Autodesk Fusion 360 part; units mm, degrees
note: some values were not read from the file. Chosen so that the rebuilt part matches the saved one: that a step has no effect.
(part 3 of 7)
  spline S620 degree 3 poles (-16.2697, 43.0639) (-16.2176, 42.4855) (-16.1655, 41.9071) (-16.1119, 41.3111) knots 0 0 0 0 1 1 1 1
  spline S621 degree 3 poles (-16.1119, 41.3111) (-16.0605, 39.9386) (-16.1203, 38.9907) (-16.5501, 37.7044) knots 0 0 0 0 1 1 1 1
  spline S622 degree 3 poles (-16.5501, 37.7044) (-16.8791, 37.7044) (-17.2082, 37.7044) (-17.5472, 37.7044) knots 0 0 0 0 1 1 1 1
  spline S623 degree 3 poles (-17.5472, 37.7044) (-17.5298, 37.2957) (-17.5125, 36.8869) (-17.4946, 36.4658) knots 0 0 0 0 1 1 1 1
  spline S624 degree 3 poles (-17.4946, 36.4658) (-17.4811, 35.9285) (-17.4676, 35.3912) (-17.4537, 34.8377) knots 0 0 0 0 1 1 1 1
  spline S625 degree 3 poles (-17.4537, 34.8377) (-17.4364, 34.3056) (-17.419, 33.7734) (-17.4011, 33.2252) knots 0 0 0 0 1 1 1 1
  spline S626 degree 3 poles (-17.4011, 33.2252) (-17.5472, 31.7217) (-17.5472, 31.7217) (-19.0429, 29.7275) knots 0 0 0 0 1 1 1 1
  spline S627 degree 3 poles (-19.0429, 29.7275) (-17.3976, 29.7275) (-15.7524, 29.7275) (-14.0573, 29.7275) knots 0 0 0 0 1 1 1 1
  spline S628 degree 3 poles (-14.0573, 29.7275) (-14.0573, 30.0565) (-14.0573, 30.3856) (-14.0573, 30.7246) knots 0 0 0 0 1 1 1 1
  spline S629 degree 3 poles (-14.0573, 30.7246) (-13.5637, 30.7246) (-13.0702, 30.7246) (-12.5616, 30.7246) knots 0 0 0 0 1 1 1 1
  spline S630 degree 3 poles (-12.5616, 30.7246) (-12.3971, 31.2182) (-12.2326, 31.7117) (-12.0631, 32.2203) knots 0 0 0 0 1 1 1 1
  spline S631 degree 3 poles (-12.0631, 32.2203) (-11.8725, 31.3946) (-11.7071, 30.5628) (-11.5645, 29.7275) knots 0 0 0 0 1 1 1 1
  spline S632 degree 3 poles (-11.5645, 29.7275) (-12.0631, 29.2289) (-12.0631, 29.2289) (-13.8567, 29.1803) knots 0 0 0 0 1 1 1 1
  spline S633 degree 3 poles (-13.8567, 29.1803) (-14.5987, 29.1836) (-15.3407, 29.1895) (-16.0827, 29.1978) knots 0 0 0 0 1 1 1 1
  spline S634 degree 3 poles (-16.0827, 29.1978) (-16.65, 29.2012) (-16.65, 29.2012) (-17.2288, 29.2046) knots 0 0 0 0 1 1 1 1
  spline S635 degree 3 poles (-17.2288, 29.2046) (-18.1659, 29.2105) (-19.1029, 29.2194) (-20.04, 29.2289) knots 0 0 0 0 1 1 1 1
  spline S636 degree 3 poles (-20.04, 29.2289) (-20.2868, 29.9693) (-20.2868, 29.9693) (-20.5385, 30.7246) knots 0 0 0 0 1 1 1 1
  spline S637 degree 3 poles (-20.5385, 30.7246) (-20.374, 31.0537) (-20.2095, 31.3827) (-20.04, 31.7217) knots 0 0 0 0 1 1 1 1
  spline S638 degree 3 poles (-20.04, 31.7217) (-19.7109, 31.7217) (-19.3819, 31.7217) (-19.0429, 31.7217) knots 0 0 0 0 1 1 1 1
  spline S639 degree 3 poles (-19.0429, 31.7217) (-18.3848, 36.4929) (-17.7267, 41.2641) (-17.0486, 46.1798) knots 0 0 0 0 1 1 1 1
  spline S640 degree 3 poles (-38.9851, 32.7188) (-37.998, 32.3898) (-37.0108, 32.0607) (-35.9938, 31.7217) knots 0 0 0 0 1 1 1 1
  spline S641 degree 3 poles (-35.9938, 31.7217) (-35.9938, 31.3927) (-35.9938, 31.0636) (-35.9938, 30.7246) knots 0 0 0 0 1 1 1 1
  spline S642 degree 3 poles (-35.9938, 30.7246) (-35.3357, 31.0537) (-34.6776, 31.3827) (-33.9995, 31.7217) knots 0 0 0 0 1 1 1 1
  spline S643 degree 3 poles (-33.9995, 31.7217) (-33.9995, 32.0508) (-33.9995, 32.3798) (-33.9995, 32.7188) knots 0 0 0 0 1 1 1 1
  spline S644 degree 3 poles (-33.9995, 32.7188) (-33.506, 32.7188) (-33.0124, 32.7188) (-32.5039, 32.7188) knots 0 0 0 0 1 1 1 1
  spline S645 degree 3 poles (-32.5039, 32.7188) (-32.3394, 32.3898) (-32.1748, 32.0607) (-32.0053, 31.7217) knots 0 0 0 0 1 1 1 1
  spline S646 degree 3 poles (-32.0053, 31.7217) (-30.5246, 31.7217) (-29.0439, 31.7217) (-27.5183, 31.7217) knots 0 0 0 0 1 1 1 1
  spline S647 degree 3 poles (-27.5183, 31.7217) (-27.3538, 31.0636) (-27.1893, 30.4055) (-27.0198, 29.7275) knots 0 0 0 0 1 1 1 1
  spline S648 degree 3 poles (-27.0198, 29.7275) (-30.4911, 28.562) (-33.1588, 28.6348) (-36.4923, 30.2261) knots 0 0 0 0 1 1 1 1
  spline S649 degree 3 poles (-36.4923, 30.2261) (-37.5065, 30.9946) (-38.1768, 31.7219) (-38.9851, 32.7188) knots 0 0 0 0 1 1 1 1
  spline S650 degree 3 poles (-5.0833, -7.6642) (-5.0833, -7.9933) (-5.0833, -8.3223) (-5.0833, -8.6613) knots 0 0 0 0 1 1 1 1
  spline S651 degree 3 poles (-5.0833, -8.6613) (-4.2607, -8.8258) (-3.4381, -8.9904) (-2.5905, -9.1599) knots 0 0 0 0 1 1 1 1
  spline S652 degree 3 poles (-2.5905, -9.1599) (-2.9196, -9.9825) (-3.2486, -10.8051) (-3.5876, -11.6527) knots 0 0 0 0 1 1 1 1
  spline S653 degree 3 poles (-3.5876, -11.6527) (-3.9, -11.6829) (-4.2123, -11.7131) (-4.5341, -11.7442) knots 0 0 0 0 1 1 1 1
  spline S654 degree 3 poles (-4.5341, -11.7442) (-4.9416, -11.786) (-5.349, -11.8277) (-5.7688, -11.8708) knots 0 0 0 0 1 1 1 1
  spline S655 degree 3 poles (-5.7688, -11.8708) (-6.1737, -11.9113) (-6.5786, -11.9517) (-6.9957, -11.9935) knots 0 0 0 0 1 1 1 1
  spline S656 degree 3 poles (-6.9957, -11.9935) (-8.0959, -12.0968) (-8.0959, -12.0968) (-9.0717, -12.6498) knots 0 0 0 0 1 1 1 1
  spline S657 degree 3 poles (-9.0717, -12.6498) (-9.4008, -12.3207) (-9.7298, -11.9917) (-10.0689, -11.6527) knots 0 0 0 0 1 1 1 1
  spline S658 degree 3 poles (-10.0689, -11.6527) (-8.8515, -8.8526) (-8.8515, -8.8526) (-7.5761, -7.9758) knots 0 0 0 0 1 1 1 1
  spline S659 degree 3 poles (-7.5761, -7.9758) (-6.579, -7.6642) (-6.579, -7.6642) (-5.0833, -7.6642) knots 0 0 0 0 1 1 1 1
  spline S660 degree 3 poles (-5.5819, 0.8112) (-5.471, 0.363) (-5.471, 0.363) (-5.3579, -0.0943) knots 0 0 0 0 1 1 1 1
  spline S661 degree 3 poles (-5.3579, -0.0943) (-5.1425, -0.9483) (-4.913, -1.7987) (-4.6782, -2.6475) knots 0 0 0 0 1 1 1 1
  spline S662 degree 3 poles (-4.6782, -2.6475) (-4.5847, -4.1743) (-4.5847, -4.1743) (-5.5195, -5.5453) knots 0 0 0 0 1 1 1 1
  spline S663 degree 3 poles (-5.5195, -5.5453) (-5.8692, -5.9155) (-6.2188, -6.2857) (-6.579, -6.6671) knots 0 0 0 0 1 1 1 1
  spline S664 degree 3 poles (-6.579, -6.6671) (-6.7435, -6.9961) (-6.908, -7.3252) (-7.0775, -7.6642) knots 0 0 0 0 1 1 1 1
  spline S665 degree 3 poles (-7.0775, -7.6642) (-8.3259, -8.0888) (-8.3259, -8.0888) (-9.8507, -8.4744) knots 0 0 0 0 1 1 1 1
  spline S666 degree 3 poles (-9.8507, -8.4744) (-10.3552, -8.6042) (-10.8597, -8.734) (-11.3795, -8.8678) knots 0 0 0 0 1 1 1 1
  spline S667 degree 3 poles (-11.3795, -8.8678) (-11.7696, -8.9642) (-12.1597, -9.0606) (-12.5616, -9.1599) knots 0 0 0 0 1 1 1 1
  spline S668 degree 3 poles (-12.5616, -9.1599) (-12.5616, -8.8308) (-12.5616, -8.5018) (-12.5616, -8.1628) knots 0 0 0 0 1 1 1 1
  spline S669 degree 3 poles (-12.5616, -8.1628) (-12.8907, -8.1628) (-13.2197, -8.1628) (-13.5588, -8.1628) knots 0 0 0 0 1 1 1 1
  spline S670 degree 3 poles (-13.5588, -8.1628) (-14.1196, -5.2961) (-14.1196, -5.2961) (-13.5588, -4.1743) knots 0 0 0 0 1 1 1 1
  spline S671 degree 3 poles (-13.5588, -4.1743) (-13.2297, -4.1743) (-12.9007, -4.1743) (-12.5616, -4.1743) knots 0 0 0 0 1 1 1 1
  spline S672 degree 3 poles (-12.5616, -4.1743) (-12.5616, -3.3517) (-12.5616, -2.5291) (-12.5616, -1.6815) knots 0 0 0 0 1 1 1 1
  spline S673 degree 3 poles (-12.5616, -1.6815) (-12.2326, -1.6815) (-11.9035, -1.6815) (-11.5645, -1.6815) knots 0 0 0 0 1 1 1 1
  spline S674 degree 3 poles (-11.5645, -1.6815) (-11.7291, -3.4913) (-11.8936, -5.301) (-12.0631, -7.1656) knots 0 0 0 0 1 1 1 1
  spline S675 degree 3 poles (-12.0631, -7.1656) (-10.5992, -7.8313) (-10.5992, -7.8313) (-9.3152, -7.1715) knots 0 0 0 0 1 1 1 1
  spline S676 degree 3 poles (-9.3152, -7.1715) (-7.7171, -5.8795) (-7.2541, -4.4864) (-6.6724, -2.5852) knots 0 0 0 0 1 1 1 1
  spline S677 degree 3 poles (-6.6724, -2.5852) (-6.5648, -2.259) (-6.4572, -1.9329) (-6.3462, -1.5968) knots 0 0 0 0 1 1 1 1
  spline S678 degree 3 poles (-6.3462, -1.5968) (-6.0834, -0.7967) (-5.8315, 0.007) (-5.5819, 0.8112) knots 0 0 0 0 1 1 1 1
  spline S679 degree 3 poles (24.3296, 14.9831) (26.0233, 14.6232) (26.8004, 13.6084) (27.8214, 12.278) knots 0 0 0 0 1 1 1 1
  spline S680 degree 3 poles (27.8214, 12.278) (28.5444, 10.1089) (28.5619, 8.1594) (27.946, 5.9526) knots 0 0 0 0 1 1 1 1
  spline S681 degree 3 poles (27.946, 5.9526) (26.9552, 4.1196) (26.0218, 3.0365) (24.0199, 2.3692) knots 0 0 0 0 1 1 1 1
  spline S682 degree 3 poles (24.0199, 2.3692) (23.6292, 2.3487) (23.2384, 2.3281) (22.8358, 2.3069) knots 0 0 0 0 1 1 1 1
  spline S683 degree 3 poles (22.8358, 2.3069) (22.5068, 2.636) (22.1777, 2.965) (21.8387, 3.304) knots 0 0 0 0 1 1 1 1
  spline S684 degree 3 poles (21.8387, 3.304) (22.6613, 3.304) (23.484, 3.304) (24.3315, 3.304) knots 0 0 0 0 1 1 1 1
  spline S685 degree 3 poles (24.3315, 3.304) (24.3624, 3.6125) (24.3932, 3.921) (24.425, 4.2388) knots 0 0 0 0 1 1 1 1
  spline S686 degree 3 poles (24.425, 4.2388) (24.5587, 4.5884) (24.6923, 4.938) (24.8301, 5.2983) knots 0 0 0 0 1 1 1 1
  spline S687 degree 3 poles (24.8301, 5.2983) (26.1018, 5.863) (26.1018, 5.863) (27.3228, 6.2954) knots 0 0 0 0 1 1 1 1
  spline S688 degree 3 poles (27.3228, 6.2954) (27.2795, 7.1891) (27.2256, 8.0823) (27.167, 8.9751) knots 0 0 0 0 1 1 1 1
  spline S689 degree 3 poles (27.167, 8.9751) (27.1237, 9.7212) (27.1237, 9.7212) (27.0794, 10.4825) knots 0 0 0 0 1 1 1 1
  spline S690 degree 3 poles (27.0794, 10.4825) (26.9952, 10.9105) (26.911, 11.3385) (26.8243, 11.7795) knots 0 0 0 0 1 1 1 1
  spline S691 degree 3 poles (26.8243, 11.7795) (26.3307, 12.1085) (25.8371, 12.4376) (25.3286, 12.7766) knots 0 0 0 0 1 1 1 1
  spline S692 degree 3 poles (25.3286, 12.7766) (25.3286, 13.1056) (25.3286, 13.4347) (25.3286, 13.7737) knots 0 0 0 0 1 1 1 1
  spline S693 degree 3 poles (25.3286, 13.7737) (24.835, 13.6092) (24.3415, 13.4447) (23.8329, 13.2751) knots 0 0 0 0 1 1 1 1
  spline S694 degree 3 poles (23.8329, 13.2751) (23.1378, 13.2419) (22.4411, 13.2326) (21.7452, 13.244) knots 0 0 0 0 1 1 1 1
  spline S695 degree 3 poles (21.7452, 13.244) (20.8044, 13.2594) (20.8044, 13.2594) (19.8445, 13.2751) knots 0 0 0 0 1 1 1 1
  spline S696 degree 3 poles (19.8445, 13.2751) (20.9861, 14.9876) (22.3538, 15.0522) (24.3296, 14.9831) knots 0 0 0 0 1 1 1 1
  spline S697 degree 3 poles (-31.5068, 15.2694) (-31.1777, 15.2694) (-30.8487, 15.2694) (-30.5097, 15.2694) knots 0 0 0 0 1 1 1 1
  spline S698 degree 3 poles (-30.5097, 15.2694) (-30.5097, 14.4468) (-30.5097, 13.6241) (-30.5097, 12.7766) knots 0 0 0 0 1 1 1 1
  spline S699 degree 3 poles (-30.5097, 12.7766) (-30.2012, 12.9411) (-29.8927, 13.1056) (-29.5749, 13.2751) knots 0 0 0 0 1 1 1 1
  spline S700 degree 3 poles (-29.5749, 13.2751) (-26.8442, 14.149) (-24.1154, 14.2507) (-21.4733, 13.0882) knots 0 0 0 0 1 1 1 1
  spline S701 degree 3 poles (-21.4733, 13.0882) (-21.1648, 12.8208) (-20.8564, 12.5535) (-20.5385, 12.278) knots 0 0 0 0 1 1 1 1
  spline S702 degree 3 poles (-20.5385, 12.278) (-20.5385, 11.949) (-20.5385, 11.6199) (-20.5385, 11.2809) knots 0 0 0 0 1 1 1 1
  spline S703 degree 3 poles (-20.5385, 11.2809) (-21.0321, 11.1164) (-21.5257, 10.9519) (-22.0342, 10.7824) knots 0 0 0 0 1 1 1 1
  spline S704 degree 3 poles (-22.0342, 10.7824) (-22.0342, 11.1114) (-22.0342, 11.4405) (-22.0342, 11.7795) knots 0 0 0 0 1 1 1 1
  spline S705 degree 3 poles (-22.0342, 11.7795) (-25.4087, 11.8301) (-28.6666, 11.7946) (-32.0053, 11.2809) knots 0 0 0 0 1 1 1 1
  spline S706 degree 3 poles (-32.0053, 11.2809) (-32.4693, 12.5801) (-32.5783, 13.0967) (-32.0365, 14.3969) knots 0 0 0 0 1 1 1 1
  spline S707 degree 3 poles (-32.0365, 14.3969) (-31.8617, 14.6848) (-31.6869, 14.9727) (-31.5068, 15.2694) knots 0 0 0 0 1 1 1 1
  spline S708 degree 3 poles (-28.0792, 48.7661) (-27.5663, 48.7732) (-27.0535, 48.7802) (-26.5251, 48.7875) knots 0 0 0 0 1 1 1 1
  spline S709 degree 3 poles (-26.5251, 48.7875) (-24.9983, 48.6705) (-23.9125, 48.3196) (-22.5328, 47.6755) knots 0 0 0 0 1 1 1 1
  spline S710 degree 3 poles (-22.5328, 47.6755) (-24.1968, 47.1208) (-24.4136, 47.2732) (-26.0227, 47.6755) knots 0 0 0 0 1 1 1 1
  spline S711 degree 3 poles (-26.0227, 47.6755) (-27.1858, 47.6949) (-28.3495, 47.6979) (-29.5125, 47.6755) knots 0 0 0 0 1 1 1 1
  spline S712 degree 3 poles (-29.5125, 47.6755) (-29.5125, 47.511) (-29.5125, 47.3465) (-29.5125, 47.177) knots 0 0 0 0 1 1 1 1
  spline S713 degree 3 poles (-29.5125, 47.177) (-28.3609, 46.8479) (-27.2092, 46.5189) (-26.0227, 46.1798) knots 0 0 0 0 1 1 1 1
  spline S714 degree 3 poles (-26.0227, 46.1798) (-26.0227, 46.0153) (-26.0227, 45.8508) (-26.0227, 45.6813) knots 0 0 0 0 1 1 1 1
  spline S715 degree 3 poles (-26.0227, 45.6813) (-26.335, 45.6684) (-26.6473, 45.6556) (-26.9691, 45.6423) knots 0 0 0 0 1 1 1 1
  spline S716 degree 3 poles (-26.9691, 45.6423) (-27.3766, 45.6141) (-27.784, 45.5858) (-28.2038, 45.5566) knots 0 0 0 0 1 1 1 1
  spline S717 degree 3 poles (-28.2038, 45.5566) (-28.6087, 45.5335) (-29.0136, 45.5104) (-29.4308, 45.4865) knots 0 0 0 0 1 1 1 1
  spline S718 degree 3 poles (-29.4308, 45.4865) (-30.5867, 45.289) (-30.5867, 45.289) (-31.1173, 44.2479) knots 0 0 0 0 1 1 1 1
  spline S719 degree 3 poles (-31.1173, 44.2479) (-31.2458, 43.8983) (-31.3743, 43.5487) (-31.5068, 43.1885) knots 0 0 0 0 1 1 1 1
  spline S720 degree 3 poles (-31.5068, 43.1885) (-31.6919, 42.7361) (-31.8769, 42.2836) (-32.0676, 41.8175) knots 0 0 0 0 1 1 1 1
  spline S721 degree 3 poles (-32.0676, 41.8175) (-32.2116, 41.4473) (-32.3556, 41.0771) (-32.5039, 40.6957) knots 0 0 0 0 1 1 1 1
  spline S722 degree 3 poles (-32.5039, 40.6957) (-33.096, 42.4055) (-32.9039, 43.3769) (-32.2858, 45.0581) knots 0 0 0 0 1 1 1 1
  spline S723 degree 3 poles (-32.2858, 45.0581) (-32.1424, 45.4565) (-31.9991, 45.855) (-31.8515, 46.2655) knots 0 0 0 0 1 1 1 1
  spline S724 degree 3 poles (-31.8515, 46.2655) (-31.6808, 46.7167) (-31.6808, 46.7167) (-31.5068, 47.177) knots 0 0 0 0 1 1 1 1
  spline S725 degree 3 poles (-31.5068, 47.177) (-32.4939, 47.0124) (-33.4811, 46.8479) (-34.4981, 46.6784) knots 0 0 0 0 1 1 1 1
  spline S726 degree 3 poles (-34.4981, 46.6784) (-32.3504, 48.3817) (-30.8035, 48.7491) (-28.0792, 48.7661) knots 0 0 0 0 1 1 1 1
  spline S727 degree 3 poles (-73.3855, 16.2665) (-72.6376, 15.581) (-72.6376, 15.581) (-71.8898, 14.7708) knots 0 0 0 0 1 1 1 1
  spline S728 degree 3 poles (-71.8898, 14.7708) (-71.8898, 14.4418) (-71.8898, 14.1127) (-71.8898, 13.7737) knots 0 0 0 0 1 1 1 1
  spline S729 degree 3 poles (-71.8898, 13.7737) (-72.2189, 13.7737) (-72.5479, 13.7737) (-72.8869, 13.7737) knots 0 0 0 0 1 1 1 1
  spline S730 degree 3 poles (-72.8869, 13.7737) (-72.964, 13.3418) (-72.964, 13.3418) (-73.0427, 12.9012) knots 0 0 0 0 1 1 1 1
  spline S731 degree 3 poles (-73.0427, 12.9012) (-73.4398, 11.6017) (-73.9791, 10.7956) (-74.8811, 9.7853) knots 0 0 0 0 1 1 1 1
  spline S732 degree 3 poles (-74.8811, 9.7853) (-75.2102, 9.7853) (-75.5392, 9.7853) (-75.8783, 9.7853) knots 0 0 0 0 1 1 1 1
  spline S733 degree 3 poles (-75.8783, 9.7853) (-75.8783, 8.9626) (-75.8783, 8.14) (-75.8783, 7.2925) knots 0 0 0 0 1 1 1 1
  spline S734 degree 3 poles (-75.8783, 7.2925) (-76.2073, 7.2925) (-76.5363, 7.2925) (-76.8754, 7.2925) knots 0 0 0 0 1 1 1 1
  spline S735 degree 3 poles (-76.8754, 7.2925) (-77.2044, 6.3053) (-77.5335, 5.3182) (-77.8725, 4.3011) knots 0 0 0 0 1 1 1 1
  spline S736 degree 3 poles (-77.8725, 4.3011) (-78.8054, 6.7198) (-77.5957, 8.5127) (-76.6164, 10.7512) knots 0 0 0 0 1 1 1 1
  spline S737 degree 3 poles (-76.6164, 10.7512) (-75.6728, 12.703) (-74.5953, 14.469) (-73.3855, 16.2665) knots 0 0 0 0 1 1 1 1
  spline S738 degree 3 poles (47.2651, -7.6642) (48.418, -7.5396) (48.418, -7.5396) (49.7579, -7.6642) knots 0 0 0 0 1 1 1 1
  spline S739 degree 3 poles (49.7579, -7.6642) (50.7238, -8.5055) (50.7238, -8.5055) (51.2535, -9.6584) knots 0 0 0 0 1 1 1 1
  spline S740 degree 3 poles (51.2535, -9.6584) (50.9731, -10.9983) (50.9731, -10.9983) (50.2564, -12.1512) knots 0 0 0 0 1 1 1 1
  spline S741 degree 3 poles (50.2564, -12.1512) (49.3216, -12.6809) (49.3216, -12.6809) (48.2622, -12.6498) knots 0 0 0 0 1 1 1 1
  spline S742 degree 3 poles (48.2622, -12.6498) (47.1404, -11.6838) (47.1404, -11.6838) (46.268, -10.6555) knots 0 0 0 0 1 1 1 1
  spline S743 degree 3 poles (46.268, -10.6555) (46.597, -9.6684) (46.9261, -8.6813) (47.2651, -7.6642) knots 0 0 0 0 1 1 1 1
  spline S744 degree 3 poles (-57.8854, 16.8799) (-56.9331, 16.765) (-56.9331, 16.765) (-55.936, 15.7679) knots 0 0 0 0 1 1 1 1
  spline S745 degree 3 poles (-55.936, 15.7679) (-55.8737, 14.4592) (-55.8737, 14.4592) (-55.936, 13.2751) knots 0 0 0 0 1 1 1 1
  spline S746 degree 3 poles (-55.936, 13.2751) (-57.0877, 13.1106) (-58.2393, 12.9461) (-59.4259, 12.7766) knots 0 0 0 0 1 1 1 1
  spline S747 degree 3 poles (-59.4259, 12.7766) (-59.2614, 13.2702) (-59.0969, 13.7637) (-58.9274, 14.2723) knots 0 0 0 0 1 1 1 1
  spline S748 degree 3 poles (-58.9274, 14.2723) (-59.75, 14.4368) (-60.5726, 14.6013) (-61.4201, 14.7708) knots 0 0 0 0 1 1 1 1
  spline S749 degree 3 poles (-61.4201, 14.7708) (-61.4201, 14.4418) (-61.4201, 14.1127) (-61.4201, 13.7737) knots 0 0 0 0 1 1 1 1
  spline S750 degree 3 poles (-61.4201, 13.7737) (-61.7492, 13.7737) (-62.0782, 13.7737) (-62.4172, 13.7737) knots 0 0 0 0 1 1 1 1
  spline S751 degree 3 poles (-62.4172, 13.7737) (-61.2918, 16.6998) (-61.1108, 16.8156) (-57.8854, 16.8799) knots 0 0 0 0 1 1 1 1
  spline S752 degree 3 poles (-67.4028, 18.7593) (-66.9092, 18.5947) (-66.4157, 18.4302) (-65.9071, 18.2607) knots 0 0 0 0 1 1 1 1
  spline S753 degree 3 poles (-65.9071, 18.2607) (-66.4817, 16.7286) (-67.146, 15.2847) (-67.9014, 13.836) knots 0 0 0 0 1 1 1 1
  spline S754 degree 3 poles (-67.9014, 13.836) (-69.616, 10.4196) (-70.1059, 7.0736) (-70.3941, 3.304) knots 0 0 0 0 1 1 1 1
  spline S755 degree 3 poles (-70.3941, 3.304) (-70.7232, 3.304) (-71.0522, 3.304) (-71.3913, 3.304) knots 0 0 0 0 1 1 1 1
  spline S756 degree 3 poles (-71.3913, 3.304) (-71.4952, 6.4979) (-71.4702, 9.2517) (-70.3941, 12.278) knots 0 0 0 0 1 1 1 1
  spline S757 degree 3 poles (-70.3941, 12.278) (-70.0651, 12.278) (-69.736, 12.278) (-69.397, 12.278) knots 0 0 0 0 1 1 1 1
  spline S758 degree 3 poles (-69.397, 12.278) (-69.4073, 12.6482) (-69.4176, 13.0184) (-69.4282, 13.3998) knots 0 0 0 0 1 1 1 1
  spline S759 degree 3 poles (-69.4282, 13.3998) (-69.4004, 14.6236) (-69.244, 15.599) (-68.8985, 16.765) knots 0 0 0 0 1 1 1 1
  spline S760 degree 3 poles (-68.8985, 16.765) (-68.4049, 16.765) (-67.9113, 16.765) (-67.4028, 16.765) knots 0 0 0 0 1 1 1 1
  spline S761 degree 3 poles (-67.4028, 16.765) (-67.4028, 17.4231) (-67.4028, 18.0812) (-67.4028, 18.7593) knots 0 0 0 0 1 1 1 1
  spline S762 degree 3 poles (-20.5385, 11.2809) (-20.374, 11.2809) (-20.2095, 11.2809) (-20.04, 11.2809) knots 0 0 0 0 1 1 1 1
  spline S763 degree 3 poles (-20.04, 11.2809) (-19.8618, 8.0442) (-20.4392, 5.5886) (-21.5356, 2.5562) knots 0 0 0 0 1 1 1 1
  spline S764 degree 3 poles (-21.5356, 2.5562) (-21.6783, 2.1462) (-21.821, 1.7361) (-21.968, 1.3137) knots 0 0 0 0 1 1 1 1
  spline S765 degree 3 poles (-21.968, 1.3137) (-22.3169, 0.3134) (-22.6734, -0.6844) (-23.0313, -1.6815) knots 0 0 0 0 1 1 1 1
  spline S766 degree 3 poles (-23.0313, -1.6815) (-24.0284, -0.6844) (-24.0284, -0.6844) (-24.1219, 0.7489) knots 0 0 0 0 1 1 1 1
  spline S767 degree 3 poles (-24.1219, 0.7489) (-24.0454, 2.024) (-23.9032, 3.0879) (-23.5299, 4.3011) knots 0 0 0 0 1 1 1 1
  spline S768 degree 3 poles (-23.5299, 4.3011) (-23.2008, 4.3011) (-22.8718, 4.3011) (-22.5328, 4.3011) knots 0 0 0 0 1 1 1 1
  spline S769 degree 3 poles (-22.5328, 4.3011) (-22.4711, 4.8667) (-22.4094, 5.4322) (-22.3458, 6.0149) knots 0 0 0 0 1 1 1 1
  spline S770 degree 3 poles (-22.3458, 6.0149) (-22.243, 6.601) (-22.1401, 7.1872) (-22.0342, 7.791) knots 0 0 0 0 1 1 1 1
  spline S771 degree 3 poles (-22.0342, 7.791) (-21.7052, 7.9556) (-21.3761, 8.1201) (-21.0371, 8.2896) knots 0 0 0 0 1 1 1 1
  spline S772 degree 3 poles (-21.0371, 8.2896) (-21.0474, 8.6906) (-21.0577, 9.0916) (-21.0683, 9.5048) knots 0 0 0 0 1 1 1 1
  spline S773 degree 3 poles (-21.0683, 9.5048) (-21.0371, 10.7824) (-21.0371, 10.7824) (-20.5385, 11.2809) knots 0 0 0 0 1 1 1 1
  spline S774 degree 3 poles (25.8272, 48.6726) (26.3207, 48.3436) (26.8143, 48.0145) (27.3228, 47.6755) knots 0 0 0 0 1 1 1 1
  spline S775 degree 3 poles (27.3228, 47.6755) (25.5131, 47.511) (23.7033, 47.3465) (21.8387, 47.177) knots 0 0 0 0 1 1 1 1
  spline S776 degree 3 poles (21.8387, 47.177) (23.0726, 46.6834) (23.0726, 46.6834) (24.3315, 46.1798) knots 0 0 0 0 1 1 1 1
  spline S777 degree 3 poles (24.3315, 46.1798) (24.3315, 46.0153) (24.3315, 45.8508) (24.3315, 45.6813) knots 0 0 0 0 1 1 1 1
  spline S778 degree 3 poles (24.3315, 45.6813) (23.3253, 45.4541) (22.3191, 45.2269) (21.3129, 44.9997) knots 0 0 0 0 1 1 1 1
  spline S779 degree 3 poles (21.3129, 44.9997) (20.2398, 44.7317) (20.2398, 44.7317) (19.3459, 43.6871) knots 0 0 0 0 1 1 1 1
  spline S780 degree 3 poles (19.3459, 43.6871) (19.3459, 44.3452) (19.3459, 45.0033) (19.3459, 45.6813) knots 0 0 0 0 1 1 1 1
  spline S781 degree 3 poles (19.3459, 45.6813) (19.8395, 45.6813) (20.3331, 45.6813) (20.8416, 45.6813) knots 0 0 0 0 1 1 1 1
  spline S782 degree 3 poles (20.8416, 45.6813) (20.2293, 46.5017) (20.2293, 46.5017) (19.3459, 47.177) knots 0 0 0 0 1 1 1 1
  spline S783 degree 3 poles (19.3459, 47.177) (18.317, 47.0132) (18.317, 47.0132) (17.3517, 46.6784) knots 0 0 0 0 1 1 1 1
  spline S784 degree 3 poles (17.3517, 46.6784) (17.0227, 46.8429) (16.6936, 47.0074) (16.3546, 47.177) knots 0 0 0 0 1 1 1 1
  spline S785 degree 3 poles (16.3546, 47.177) (19.2337, 49.1512) (22.4334, 49.0215) (25.8272, 48.6726) knots 0 0 0 0 1 1 1 1
  spline S786 degree 3 poles (-63.9129, 23.7448) (-63.5839, 23.2513) (-63.2548, 22.7577) (-62.9158, 22.2492) knots 0 0 0 0 1 1 1 1
  spline S787 degree 3 poles (-62.9158, 22.2492) (-63.3065, 21.8687) (-63.6973, 21.4882) (-64.0999, 21.0962) knots 0 0 0 0 1 1 1 1
  spline S788 degree 3 poles (-64.0999, 21.0962) (-65.4448, 19.8018) (-65.4448, 19.8018) (-66.4057, 18.2607) knots 0 0 0 0 1 1 1 1
  spline S789 degree 3 poles (-66.4057, 18.2607) (-66.7347, 18.4252) (-67.0638, 18.5898) (-67.4028, 18.7593) knots 0 0 0 0 1 1 1 1
  spline S790 degree 3 poles (-67.4028, 18.7593) (-67.5673, 18.2657) (-67.7318, 17.7721) (-67.9014, 17.2636) knots 0 0 0 0 1 1 1 1
  spline S791 degree 3 poles (-67.9014, 17.2636) (-68.0659, 17.5926) (-68.2304, 17.9217) (-68.3999, 18.2607) knots 0 0 0 0 1 1 1 1
  spline S792 degree 3 poles (-68.3999, 18.2607) (-68.729, 18.4252) (-69.058, 18.5898) (-69.397, 18.7593) knots 0 0 0 0 1 1 1 1
  spline S793 degree 3 poles (-69.397, 18.7593) (-68.7738, 20.2238) (-68.7738, 20.2238) (-67.9014, 21.7506) knots 0 0 0 0 1 1 1 1
  spline S794 degree 3 poles (-67.9014, 21.7506) (-66.9354, 22.0934) (-66.9354, 22.0934) (-65.9071, 22.2492) knots 0 0 0 0 1 1 1 1
  spline S795 degree 3 poles (-65.9071, 22.2492) (-64.8067, 22.991) (-64.8067, 22.991) (-63.9129, 23.7448) knots 0 0 0 0 1 1 1 1
  spline S796 degree 3 poles (-23.8103, 26.8296) (-21.8826, 26.7282) (-20.1085, 26.3788) (-18.2288, 25.9572) knots 0 0 0 0 1 1 1 1
  spline S797 degree 3 poles (-18.2288, 25.9572) (-16.9218, 25.6786) (-16.9218, 25.6786) (-15.0544, 25.739) knots 0 0 0 0 1 1 1 1
  spline S798 degree 3 poles (-15.0544, 25.739) (-15.0544, 25.41) (-15.0544, 25.081) (-15.0544, 24.7419) knots 0 0 0 0 1 1 1 1
  spline S799 degree 3 poles (-15.0544, 24.7419) (-16.2697, 24.7285) (-17.4848, 24.7186) (-18.7001, 24.7108) knots 0 0 0 0 1 1 1 1
  spline S800 degree 3 poles (-18.7001, 24.7108) (-19.0443, 24.7066) (-19.3884, 24.7024) (-19.743, 24.6981) knots 0 0 0 0 1 1 1 1
  spline S801 degree 3 poles (-19.743, 24.6981) (-21.3105, 24.6905) (-22.5299, 24.741) (-24.0284, 25.2405) knots 0 0 0 0 1 1 1 1
  spline S802 degree 3 poles (-24.0284, 25.2405) (-24.0284, 24.7469) (-24.0284, 24.2534) (-24.0284, 23.7448) knots 0 0 0 0 1 1 1 1
  spline S803 degree 3 poles (-24.0284, 23.7448) (-23.6994, 23.7448) (-23.3703, 23.7448) (-23.0313, 23.7448) knots 0 0 0 0 1 1 1 1
  spline S804 degree 3 poles (-23.0313, 23.7448) (-23.0313, 23.4158) (-23.0313, 23.0867) (-23.0313, 22.7477) knots 0 0 0 0 1 1 1 1
  spline S805 degree 3 poles (-23.0313, 22.7477) (-24.2652, 23.2413) (-24.2652, 23.2413) (-25.5241, 23.7448) knots 0 0 0 0 1 1 1 1
  spline S806 degree 3 poles (-25.5241, 23.7448) (-25.5454, 24.5755) (-25.5444, 25.4069) (-25.5241, 26.2376) knots 0 0 0 0 1 1 1 1
  spline S807 degree 3 poles (-25.5241, 26.2376) (-25.0255, 26.7362) (-25.0255, 26.7362) (-23.8103, 26.8296) knots 0 0 0 0 1 1 1 1
  spline S808 degree 3 poles (-45.4663, 24.7419) (-43.3459, 22.7889) (-42.1288, 21.316) (-41.844, 18.4009) knots 0 0 0 0 1 1 1 1
  spline S809 degree 3 poles (-41.844, 18.4009) (-41.8466, 17.9433) (-41.8492, 17.4858) (-41.8518, 17.0143) knots 0 0 0 0 1 1 1 1
  spline S810 degree 3 poles (-41.8518, 17.0143) (-41.8492, 16.5567) (-41.8467, 16.0992) (-41.844, 15.6277) knots 0 0 0 0 1 1 1 1
  spline S811 degree 3 poles (-41.844, 15.6277) (-41.9851, 14.1836) (-42.3735, 13.0938) (-42.9736, 11.7795) knots 0 0 0 0 1 1 1 1
  spline S812 degree 3 poles (-42.9736, 11.7795) (-43.1381, 11.7795) (-43.3026, 11.7795) (-43.4721, 11.7795) knots 0 0 0 0 1 1 1 1
  spline S813 degree 3 poles (-43.4721, 11.7795) (-43.4855, 12.8389) (-43.4952, 13.8983) (-43.5033, 14.9578) knots 0 0 0 0 1 1 1 1
  spline S814 degree 3 poles (-43.5033, 14.9578) (-43.5091, 15.5477) (-43.5148, 16.1377) (-43.5208, 16.7456) knots 0 0 0 0 1 1 1 1
  spline S815 degree 3 poles (-43.5208, 16.7456) (-43.4721, 18.2607) (-43.4721, 18.2607) (-42.9736, 19.2578) knots 0 0 0 0 1 1 1 1
  spline S816 degree 3 poles (-42.9736, 19.2578) (-43.2101, 19.556) (-43.4466, 19.8542) (-43.6902, 20.1615) knots 0 0 0 0 1 1 1 1
  spline S817 degree 3 poles (-43.6902, 20.1615) (-44.4692, 21.252) (-44.4692, 21.252) (-44.9678, 22.7477) knots 0 0 0 0 1 1 1 1
  spline S818 degree 3 poles (-44.9678, 22.7477) (-45.4614, 22.5832) (-45.9549, 22.4187) (-46.4635, 22.2492) knots 0 0 0 0 1 1 1 1
  spline S819 degree 3 poles (-46.4635, 22.2492) (-46.628, 22.5782) (-46.7925, 22.9072) (-46.962, 23.2463) knots 0 0 0 0 1 1 1 1
  spline S820 degree 3 poles (-46.962, 23.2463) (-46.633, 23.2463) (-46.3039, 23.2463) (-45.9649, 23.2463) knots 0 0 0 0 1 1 1 1
  spline S821 degree 3 poles (-45.9649, 23.2463) (-45.8004, 23.7398) (-45.6358, 24.2334) (-45.4663, 24.7419) knots 0 0 0 0 1 1 1 1
  spline S822 degree 3 poles (-24.0284, 25.2405) (-21.067, 25.076) (-18.1056, 24.9114) (-15.0544, 24.7419) knots 0 0 0 0 1 1 1 1
  spline S823 degree 3 poles (-15.0544, 24.7419) (-17.0486, 22.7477) (-17.0486, 22.7477) (-18.5521, 22.553) knots 0 0 0 0 1 1 1 1
  spline S824 degree 3 poles (-18.5521, 22.553) (-19.0842, 22.5761) (-19.6164, 22.5992) (-20.1646, 22.6231) knots 0 0 0 0 1 1 1 1
  spline S825 degree 3 poles (-20.1646, 22.6231) (-20.7019, 22.6411) (-21.2392, 22.6591) (-21.7927, 22.6776) knots 0 0 0 0 1 1 1 1
  spline S826 degree 3 poles (-21.7927, 22.6776) (-22.2015, 22.7007) (-22.6102, 22.7239) (-23.0313, 22.7477) knots 0 0 0 0 1 1 1 1
  spline S827 degree 3 poles (-23.0313, 22.7477) (-23.0313, 23.0768) (-23.0313, 23.4058) (-23.0313, 23.7448) knots 0 0 0 0 1 1 1 1
  spline S828 degree 3 poles (-23.0313, 23.7448) (-23.3604, 23.7448) (-23.6894, 23.7448) (-24.0284, 23.7448) knots 0 0 0 0 1 1 1 1
  spline S829 degree 3 poles (-24.0284, 23.7448) (-24.0284, 24.2384) (-24.0284, 24.732) (-24.0284, 25.2405) knots 0 0 0 0 1 1 1 1
  spline S830 degree 3 poles (31.8098, 33.2174) (34.081, 32.9404) (34.081, 32.9404) (34.8012, 32.2203) knots 0 0 0 0 1 1 1 1
  spline S831 degree 3 poles (34.8012, 32.2203) (34.9258, 31.005) (34.9258, 31.005) (34.8012, 29.7275) knots 0 0 0 0 1 1 1 1
  spline S832 degree 3 poles (34.8012, 29.7275) (33.3055, 28.7304) (33.3055, 28.7304) (32.2772, 28.855) knots 0 0 0 0 1 1 1 1
  spline S833 degree 3 poles (32.2772, 28.855) (31.3113, 29.2289) (31.3113, 29.2289) (30.3142, 30.2261) knots 0 0 0 0 1 1 1 1
  spline S834 degree 3 poles (30.3142, 30.2261) (30.4971, 31.6891) (30.7451, 32.1527) (31.8098, 33.2174) knots 0 0 0 0 1 1 1 1
  spline S835 degree 3 poles (-27.5183, 25.2405) (-27.6828, 24.7469) (-27.8474, 24.2534) (-28.0169, 23.7448) knots 0 0 0 0 1 1 1 1
  spline S836 degree 3 poles (-28.0169, 23.7448) (-28.0169, 24.0739) (-28.0169, 24.4029) (-28.0169, 24.7419) knots 0 0 0 0 1 1 1 1
  spline S837 degree 3 poles (-28.0169, 24.7419) (-29.532, 24.4813) (-29.532, 24.4813) (-30.6655, 23.4955) knots 0 0 0 0 1 1 1 1
  spline S838 degree 3 poles (-30.6655, 23.4955) (-31.9543, 22.3499) (-33.3255, 22.4068) (-34.9967, 22.2492) knots 0 0 0 0 1 1 1 1
  spline S839 degree 3 poles (-34.9967, 22.2492) (-35.1612, 21.7556) (-35.3257, 21.262) (-35.4952, 20.7535) knots 0 0 0 0 1 1 1 1
  spline S840 degree 3 poles (-35.4952, 20.7535) (-35.9888, 20.7535) (-36.4824, 20.7535) (-36.9909, 20.7535) knots 0 0 0 0 1 1 1 1
  spline S841 degree 3 poles (-36.9909, 20.7535) (-36.9909, 21.5761) (-36.9909, 22.3987) (-36.9909, 23.2463) knots 0 0 0 0 1 1 1 1
  spline S842 degree 3 poles (-36.9909, 23.2463) (-35.6941, 23.6775) (-34.3959, 24.1024) (-33.0959, 24.5238) knots 0 0 0 0 1 1 1 1
  spline S843 degree 3 poles (-33.0959, 24.5238) (-32.728, 24.6469) (-32.3601, 24.77) (-31.981, 24.8968) knots 0 0 0 0 1 1 1 1
  spline S844 degree 3 poles (-31.981, 24.8968) (-29.1834, 25.7955) (-29.1834, 25.7955) (-27.5183, 25.2405) knots 0 0 0 0 1 1 1 1
  spline S845 degree 3 poles (51.2535, 14.7708) (50.9817, 11.2375) (49.9527, 8.1261) (48.7607, 4.7997) knots 0 0 0 0 1 1 1 1
  spline S846 degree 3 poles (48.7607, 4.7997) (48.5946, 5.4644) (48.4284, 6.1292) (48.2622, 6.7939) knots 0 0 0 0 1 1 1 1
  spline S847 degree 3 poles (48.2622, 6.7939) (48.1549, 7.1101) (48.0475, 7.4263) (47.937, 7.7521) knots 0 0 0 0 1 1 1 1
  spline S848 degree 3 poles (47.937, 7.7521) (47.7047, 9.1407) (48.0429, 10.0758) (48.4803, 11.4056) knots 0 0 0 0 1 1 1 1
  spline S849 degree 3 poles (48.4803, 11.4056) (48.6236, 11.8503) (48.7669, 12.295) (48.9146, 12.7532) knots 0 0 0 0 1 1 1 1
  spline S850 degree 3 poles (48.9146, 12.7532) (49.0284, 13.09) (49.1421, 13.4267) (49.2593, 13.7737) knots 0 0 0 0 1 1 1 1
  spline S851 degree 3 poles (49.2593, 13.7737) (48.9303, 13.9382) (48.6012, 14.1028) (48.2622, 14.2723) knots 0 0 0 0 1 1 1 1
  spline S852 degree 3 poles (48.2622, 14.2723) (49.7579, 14.7708) (49.7579, 14.7708) (51.2535, 14.7708) knots 0 0 0 0 1 1 1 1
  spline S853 degree 3 poles (-44.4692, 11.7795) (-44.1402, 11.7795) (-43.8111, 11.7795) (-43.4721, 11.7795) knots 0 0 0 0 1 1 1 1
  spline S854 degree 3 poles (-43.4721, 11.7795) (-44.316, 8.5916) (-46.8333, 6.9576) (-49.5483, 5.3606) knots 0 0 0 0 1 1 1 1
  spline S855 degree 3 poles (-49.5483, 5.3606) (-50.9505, 4.7997) (-50.9505, 4.7997) (-52.9447, 4.7997) knots 0 0 0 0 1 1 1 1
  spline S856 degree 3 poles (-52.9447, 4.7997) (-52.9447, 5.1287) (-52.9447, 5.4578) (-52.9447, 5.7968) knots 0 0 0 0 1 1 1 1
  spline S857 degree 3 poles (-52.9447, 5.7968) (-51.9575, 5.7968) (-50.9704, 5.7968) (-49.9533, 5.7968) knots 0 0 0 0 1 1 1 1
  spline S858 degree 3 poles (-49.9533, 5.7968) (-49.9533, 6.1259) (-49.9533, 6.4549) (-49.9533, 6.7939) knots 0 0 0 0 1 1 1 1
  spline S859 degree 3 poles (-49.9533, 6.7939) (-49.6243, 6.9584) (-49.2952, 7.123) (-48.9562, 7.2925) knots 0 0 0 0 1 1 1 1
  spline S860 degree 3 poles (-48.9562, 7.2925) (-48.9562, 7.786) (-48.9562, 8.2796) (-48.9562, 8.7881) knots 0 0 0 0 1 1 1 1
  spline S861 degree 3 poles (-48.9562, 8.7881) (-48.6272, 8.7881) (-48.2981, 8.7881) (-47.9591, 8.7881) knots 0 0 0 0 1 1 1 1
  spline S862 degree 3 poles (-47.9591, 8.7881) (-47.7946, 9.1172) (-47.6301, 9.4462) (-47.4606, 9.7853) knots 0 0 0 0 1 1 1 1
  spline S863 degree 3 poles (-47.4606, 9.7853) (-46.4193, 10.1212) (-45.5642, 10.2838) (-44.4692, 10.2838) knots 0 0 0 0 1 1 1 1
  spline S864 degree 3 poles (-44.4692, 10.2838) (-44.4692, 10.7774) (-44.4692, 11.271) (-44.4692, 11.7795) knots 0 0 0 0 1 1 1 1
  spline S865 degree 3 poles (-45.9649, -7.6642) (-45.6358, -8.1578) (-45.3068, -8.6513) (-44.9678, -9.1599) knots 0 0 0 0 1 1 1 1
  spline S866 degree 3 poles (-44.9678, -9.1599) (-45.4614, -9.4067) (-45.4614, -9.4067) (-45.9649, -9.6584) knots 0 0 0 0 1 1 1 1
  spline S867 degree 3 poles (-45.9649, -9.6584) (-46.0369, -9.9875) (-46.1089, -10.3165) (-46.183, -10.6555) knots 0 0 0 0 1 1 1 1
  spline S868 degree 3 poles (-46.183, -10.6555) (-46.2756, -10.9846) (-46.3681, -11.3136) (-46.4635, -11.6527) knots 0 0 0 0 1 1 1 1
  spline S869 degree 3 poles (-46.4635, -11.6527) (-46.957, -11.8172) (-47.4506, -11.9817) (-47.9591, -12.1512) knots 0 0 0 0 1 1 1 1
  spline S870 degree 3 poles (-47.9591, -12.1512) (-48.1236, -12.4803) (-48.2882, -12.8093) (-48.4577, -13.1483) knots 0 0 0 0 1 1 1 1
  spline S871 degree 3 poles (-48.4577, -13.1483) (-45.1672, -13.1483) (-41.8767, -13.1483) (-38.4866, -13.1483) knots 0 0 0 0 1 1 1 1
  spline S872 degree 3 poles (-38.4866, -13.1483) (-38.6511, -11.6676) (-38.8156, -10.1869) (-38.9851, -8.6613) knots 0 0 0 0 1 1 1 1
  spline S873 degree 3 poles (-38.9851, -8.6613) (-38.8206, -8.6613) (-38.6561, -8.6613) (-38.4866, -8.6613) knots 0 0 0 0 1 1 1 1
  spline S874 degree 3 poles (-38.4866, -8.6613) (-38.3065, -9.3979) (-38.1307, -10.1356) (-37.9568, -10.8737) knots 0 0 0 0 1 1 1 1
  spline S875 degree 3 poles (-37.9568, -10.8737) (-37.8093, -11.4897) (-37.8093, -11.4897) (-37.6589, -12.1181) knots 0 0 0 0 1 1 1 1
  spline S876 degree 3 poles (-37.6589, -12.1181) (-37.603, -12.4581) (-37.547, -12.798) (-37.4894, -13.1483) knots 0 0 0 0 1 1 1 1
  spline S877 degree 3 poles (-37.4894, -13.1483) (-37.988, -13.6469) (-37.988, -13.6469) (-39.0514, -13.7035) knots 0 0 0 0 1 1 1 1
  spline S878 degree 3 poles (-39.0514, -13.7035) (-39.5083, -13.7009) (-39.9652, -13.6983) (-40.436, -13.6956) knots 0 0 0 0 1 1 1 1
  spline S879 degree 3 poles (-40.436, -13.6956) (-40.9292, -13.694) (-41.4225, -13.6924) (-41.9307, -13.6907) knots 0 0 0 0 1 1 1 1
  spline S880 degree 3 poles (-41.9307, -13.6907) (-42.4496, -13.6865) (-42.9686, -13.6823) (-43.5033, -13.678) knots 0 0 0 0 1 1 1 1
  spline S881 degree 3 poles (-43.5033, -13.678) (-44.0242, -13.6758) (-44.545, -13.6735) (-45.0817, -13.6712) knots 0 0 0 0 1 1 1 1
  spline S882 degree 3 poles (-45.0817, -13.6712) (-46.3732, -13.6653) (-47.6647, -13.6571) (-48.9562, -13.6469) knots 0 0 0 0 1 1 1 1
  spline S883 degree 3 poles (-48.9562, -13.6469) (-48.9562, -11.4659) (-48.7549, -11.1517) (-47.4606, -9.5338) knots 0 0 0 0 1 1 1 1
  spline S884 degree 3 poles (-47.4606, -9.5338) (-47.1829, -9.1816) (-46.9053, -8.8294) (-46.6192, -8.4666) knots 0 0 0 0 1 1 1 1
  spline S885 degree 3 poles (-46.6192, -8.4666) (-46.4033, -8.2018) (-46.1874, -7.937) (-45.9649, -7.6642) knots 0 0 0 0 1 1 1 1
  spline S886 degree 3 poles (-30.0111, 24.7419) (-29.353, 24.7419) (-28.6949, 24.7419) (-28.0169, 24.7419) knots 0 0 0 0 1 1 1 1
  spline S887 degree 3 poles (-28.0169, 24.7419) (-28.074, 24.0248) (-28.1376, 23.3082) (-28.2038, 22.5919) knots 0 0 0 0 1 1 1 1
  spline S888 degree 3 poles (-28.2038, 22.5919) (-28.2385, 22.1928) (-28.2732, 21.7937) (-28.309, 21.3825) knots 0 0 0 0 1 1 1 1
  spline S889 degree 3 poles (-28.309, 21.3825) (-28.5154, 20.2549) (-28.5154, 20.2549) (-29.5125, 18.7593) knots 0 0 0 0 1 1 1 1
  spline S890 degree 3 poles (-29.5125, 18.7593) (-29.5125, 19.2528) (-29.5125, 19.7464) (-29.5125, 20.2549) knots 0 0 0 0 1 1 1 1
  spline S891 degree 3 poles (-29.5125, 20.2549) (-30.3352, 20.4195) (-31.1578, 20.584) (-32.0053, 20.7535) knots 0 0 0 0 1 1 1 1
  spline S892 degree 3 poles (-32.0053, 20.7535) (-31.8408, 21.5761) (-31.6763, 22.3987) (-31.5068, 23.2463) knots 0 0 0 0 1 1 1 1
  spline S893 degree 3 poles (-31.5068, 23.2463) (-31.1777, 23.2463) (-30.8487, 23.2463) (-30.5097, 23.2463) knots 0 0 0 0 1 1 1 1
  spline S894 degree 3 poles (-30.5097, 23.2463) (-30.3451, 23.7398) (-30.1806, 24.2334) (-30.0111, 24.7419) knots 0 0 0 0 1 1 1 1
  spline S895 degree 3 poles (7.8792, 42.1914) (8.0437, 42.1914) (8.2082, 42.1914) (8.3777, 42.1914) knots 0 0 0 0 1 1 1 1
  spline S896 degree 3 poles (8.3777, 42.1914) (8.0794, 38.1995) (7.756, 34.2115) (7.3806, 30.2261) knots 0 0 0 0 1 1 1 1
  spline S897 degree 3 poles (7.3806, 30.2261) (6.3935, 30.5551) (5.4063, 30.8841) (4.3893, 31.2232) knots 0 0 0 0 1 1 1 1
  spline S898 degree 3 poles (4.3893, 31.2232) (4.6132, 31.962) (4.8427, 32.6992) (5.0748, 33.4355) knots 0 0 0 0 1 1 1 1
  spline S899 degree 3 poles (5.0748, 33.4355) (5.202, 33.8462) (5.3293, 34.2568) (5.4604, 34.6799) knots 0 0 0 0 1 1 1 1
  spline S900 degree 3 poles (5.4604, 34.6799) (5.8849, 35.7102) (5.8849, 35.7102) (6.882, 36.2087) knots 0 0 0 0 1 1 1 1
  spline S901 degree 3 poles (6.882, 36.2087) (7.2272, 37.6096) (7.2272, 37.6096) (7.4429, 39.2312) knots 0 0 0 0 1 1 1 1
  spline S902 degree 3 poles (7.4429, 39.2312) (7.5265, 39.782) (7.61, 40.3328) (7.6961, 40.9002) knots 0 0 0 0 1 1 1 1
  spline S903 degree 3 poles (7.6961, 40.9002) (7.7565, 41.3263) (7.8169, 41.7524) (7.8792, 42.1914) knots 0 0 0 0 1 1 1 1
  spline S904 degree 3 poles (-29.014, 5.7968) (-28.8495, 5.7968) (-28.6849, 5.7968) (-28.5154, 5.7968) knots 0 0 0 0 1 1 1 1
  spline S905 degree 3 poles (-28.5154, 5.7968) (-28.9168, 2.7868) (-29.4551, -0.1922) (-30.0111, -3.1772) knots 0 0 0 0 1 1 1 1
  spline S906 degree 3 poles (-30.0111, -3.1772) (-30.3401, -3.1772) (-30.6692, -3.1772) (-31.0082, -3.1772) knots 0 0 0 0 1 1 1 1
  spline S907 degree 3 poles (-31.0082, -3.1772) (-30.9774, -3.7222) (-30.9465, -4.2672) (-30.9147, -4.8287) knots 0 0 0 0 1 1 1 1
  spline S908 degree 3 poles (-30.9147, -4.8287) (-31.0082, -6.6671) (-31.0082, -6.6671) (-31.6937, -7.5707) knots 0 0 0 0 1 1 1 1
  spline S909 degree 3 poles (-31.6937, -7.5707) (-31.9611, -7.7661) (-32.2284, -7.9615) (-32.5039, -8.1628) knots 0 0 0 0 1 1 1 1
  spline S910 degree 3 poles (-32.5039, -8.1628) (-32.8329, -8.4918) (-33.162, -8.8209) (-33.501, -9.1599) knots 0 0 0 0 1 1 1 1
  spline S911 degree 3 poles (-33.501, -9.1599) (-33.2015, -7.1076) (-32.7463, -5.2224) (-32.0813, -3.259) knots 0 0 0 0 1 1 1 1
  spline S912 degree 3 poles (-32.0813, -3.259) (-31.8138, -2.4637) (-31.8138, -2.4637) (-31.5409, -1.6523) knots 0 0 0 0 1 1 1 1
  spline S913 degree 3 poles (-31.5409, -1.6523) (-31.2618, -0.8339) (-31.2618, -0.8339) (-30.9771, 0.0011) knots 0 0 0 0 1 1 1 1
  spline S914 degree 3 poles (-30.9771, 0.0011) (-30.6951, 0.8369) (-30.6951, 0.8369) (-30.4074, 1.6896) knots 0 0 0 0 1 1 1 1
  spline S915 degree 3 poles (-30.4074, 1.6896) (-29.945, 3.0593) (-29.4804, 4.4284) (-29.014, 5.7968) knots 0 0 0 0 1 1 1 1
  spline S916 degree 3 poles (-45.9649, -0.6844) (-45.6358, -0.8489) (-45.3068, -1.0135) (-44.9678, -1.183) knots 0 0 0 0 1 1 1 1
  spline S917 degree 3 poles (-44.9678, -1.183) (-45.2132, -3.9442) (-45.2132, -3.9442) (-46.4946, -5.1091) knots 0 0 0 0 1 1 1 1
  spline S918 degree 3 poles (-46.4946, -5.1091) (-46.8134, -5.2942) (-47.1321, -5.4793) (-47.4606, -5.67) knots 0 0 0 0 1 1 1 1
  spline S919 degree 3 poles (-47.4606, -5.67) (-47.7896, -5.1764) (-48.1187, -4.6828) (-48.4577, -4.1743) knots 0 0 0 0 1 1 1 1
  spline S920 degree 3 poles (-48.4577, -4.1743) (-49.7458, -4.0495) (-49.7458, -4.0495) (-50.9505, -4.1743) knots 0 0 0 0 1 1 1 1
  spline S921 degree 3 poles (-50.9505, -4.1743) (-49.3621, -2.8582) (-47.8047, -1.6292) (-45.9649, -0.6844) knots 0 0 0 0 1 1 1 1
  spline S922 degree 3 poles (31.8098, 1.3098) (33.0438, 1.063) (33.0438, 1.063) (34.3026, 0.8112) knots 0 0 0 0 1 1 1 1
  spline S923 degree 3 poles (34.3026, 0.8112) (34.2364, 0.5278) (34.1702, 0.2444) (34.102, -0.0476) knots 0 0 0 0 1 1 1 1
  spline S924 degree 3 poles (34.102, -0.0476) (33.5605, -2.4152) (33.1145, -4.7565) (32.807, -7.1656) knots 0 0 0 0 1 1 1 1
  spline S925 degree 3 poles (32.807, -7.1656) (33.465, -7.6592) (34.1231, -8.1528) (34.8012, -8.6613) knots 0 0 0 0 1 1 1 1
  spline S926 degree 3 poles (34.8012, -8.6613) (32.3707, -8.2251) (32.3707, -8.2251) (31.8098, -7.6642) knots 0 0 0 0 1 1 1 1
  spline S927 degree 3 poles (31.8098, -7.6642) (31.8547, -6.6551) (31.9327, -5.6473) (32.028, -4.6417) knots 0 0 0 0 1 1 1 1
  spline S928 degree 3 poles (32.028, -4.6417) (32.0787, -4.0909) (32.1295, -3.5402) (32.1818, -2.9727) knots 0 0 0 0 1 1 1 1
  spline S929 degree 3 poles (32.1818, -2.9727) (32.2236, -2.5466) (32.2654, -2.1205) (32.3084, -1.6815) knots 0 0 0 0 1 1 1 1
  spline S930 degree 3 poles (32.3084, -1.6815) (32.1439, -1.6815) (31.9794, -1.6815) (31.8098, -1.6815) knots 0 0 0 0 1 1 1 1
  spline S931 degree 3 poles (31.8098, -1.6815) (31.8098, -0.6944) (31.8098, 0.2927) (31.8098, 1.3098) knots 0 0 0 0 1 1 1 1
  spline S932 degree 3 poles (11.369, -4.6729) (11.6981, -4.6729) (12.0271, -4.6729) (12.3662, -4.6729) knots 0 0 0 0 1 1 1 1
  spline S933 degree 3 poles (12.3662, -4.6729) (12.2884, -4.9679) (12.2106, -5.2628) (12.1305, -5.5668) knots 0 0 0 0 1 1 1 1
  spline S934 degree 3 poles (12.1305, -5.5668) (11.5849, -7.7817) (11.2276, -9.4126) (11.8676, -11.6527) knots 0 0 0 0 1 1 1 1
  spline S935 degree 3 poles (11.8676, -11.6527) (11.8676, -12.3107) (11.8676, -12.9688) (11.8676, -13.6469) knots 0 0 0 0 1 1 1 1
  spline S936 degree 3 poles (11.8676, -13.6469) (9.5643, -13.6469) (7.2609, -13.6469) (4.8878, -13.6469) knots 0 0 0 0 1 1 1 1
  spline S937 degree 3 poles (4.8878, -13.6469) (4.8878, -13.4824) (4.8878, -13.3178) (4.8878, -13.1483) knots 0 0 0 0 1 1 1 1
  spline S938 degree 3 poles (4.8878, -13.1483) (7.0266, -13.1483) (9.1654, -13.1483) (11.369, -13.1483) knots 0 0 0 0 1 1 1 1
  spline S939 degree 3 poles (11.369, -13.1483) (11.04, -12.6548) (10.711, -12.1612) (10.3719, -11.6527) knots 0 0 0 0 1 1 1 1
  spline S940 degree 3 poles (10.3719, -11.6527) (10.2395, -10.4861) (10.2395, -10.4861) (10.2473, -9.191) knots 0 0 0 0 1 1 1 1
  spline S941 degree 3 poles (10.2473, -9.191) (10.2447, -8.7649) (10.2422, -8.3389) (10.2395, -7.8999) knots 0 0 0 0 1 1 1 1
  spline S942 degree 3 poles (10.2395, -7.8999) (10.3783, -6.6074) (10.7176, -5.7871) (11.369, -4.6729) knots 0 0 0 0 1 1 1 1
  spline S943 degree 3 poles (-74.3826, -10.157) (-72.9292, -10.6924) (-72.0004, -11.0435) (-70.8927, -12.1512) knots 0 0 0 0 1 1 1 1
  spline S944 degree 3 poles (-70.8927, -12.1512) (-69.5341, -12.6041) (-68.5882, -12.7413) (-67.1788, -12.8075) knots 0 0 0 0 1 1 1 1
  spline S945 degree 3 poles (-67.1788, -12.8075) (-66.7563, -12.8284) (-66.3337, -12.8493) (-65.8984, -12.8708) knots 0 0 0 0 1 1 1 1
  spline S946 degree 3 poles (-65.8984, -12.8708) (-65.4591, -12.8904) (-65.0198, -12.91) (-64.5673, -12.9302) knots 0 0 0 0 1 1 1 1
  spline S947 degree 3 poles (-64.5673, -12.9302) (-63.8997, -12.9625) (-63.8997, -12.9625) (-63.2186, -12.9954) knots 0 0 0 0 1 1 1 1
  spline S948 degree 3 poles (-63.2186, -12.9954) (-62.1207, -13.0483) (-61.0226, -13.0992) (-59.9245, -13.1483) knots 0 0 0 0 1 1 1 1
  spline S949 degree 3 poles (-59.9245, -13.1483) (-59.9245, -13.3128) (-59.9245, -13.4774) (-59.9245, -13.6469) knots 0 0 0 0 1 1 1 1
  spline S950 degree 3 poles (-59.9245, -13.6469) (-61.5758, -13.7056) (-63.2268, -13.7405) (-64.8789, -13.7715) knots 0 0 0 0 1 1 1 1
  spline S951 degree 3 poles (-64.8789, -13.7715) (-65.3406, -13.7882) (-65.8024, -13.8049) (-66.2781, -13.8222) knots 0 0 0 0 1 1 1 1
  spline S952 degree 3 poles (-66.2781, -13.8222) (-69.5909, -13.8686) (-71.9762, -13.2454) (-74.8811, -11.6527) knots 0 0 0 0 1 1 1 1
  spline S953 degree 3 poles (-74.8811, -11.6527) (-74.7166, -11.1591) (-74.5521, -10.6655) (-74.3826, -10.157) knots 0 0 0 0 1 1 1 1
  spline S954 degree 3 poles (-59.4259, 17.7622) (-56.2225, 18.0039) (-56.2225, 18.0039) (-54.9389, 16.9208) knots 0 0 0 0 1 1 1 1
  spline S955 degree 3 poles (-54.9389, 16.9208) (-54.3058, 15.4569) (-54.4393, 14.7738) (-54.9389, 13.2751) knots 0 0 0 0 1 1 1 1
  spline S956 degree 3 poles (-54.9389, 13.2751) (-55.4325, 12.5348) (-55.4325, 12.5348) (-55.936, 11.7795) knots 0 0 0 0 1 1 1 1
  spline S957 degree 3 poles (-55.936, 11.7795) (-56.2651, 11.7795) (-56.5941, 11.7795) (-56.9331, 11.7795) knots 0 0 0 0 1 1 1 1
  spline S958 degree 3 poles (-56.9331, 11.7795) (-57.0976, 12.273) (-57.2622, 12.7666) (-57.4317, 13.2751) knots 0 0 0 0 1 1 1 1
  spline S959 degree 3 poles (-57.4317, 13.2751) (-56.9381, 13.2751) (-56.4445, 13.2751) (-55.936, 13.2751) knots 0 0 0 0 1 1 1 1
  spline S960 degree 3 poles (-55.936, 13.2751) (-56.2651, 14.2623) (-56.5941, 15.2494) (-56.9331, 16.2665) knots 0 0 0 0 1 1 1 1
  spline S961 degree 3 poles (-56.9331, 16.2665) (-58.4138, 16.5133) (-58.4138, 16.5133) (-59.9245, 16.765) knots 0 0 0 0 1 1 1 1
  spline S962 degree 3 poles (-59.9245, 16.765) (-59.7599, 17.0941) (-59.5954, 17.4231) (-59.4259, 17.7622) knots 0 0 0 0 1 1 1 1
  spline S963 degree 3 poles (-47.9591, 22.7477) (-47.6301, 22.7477) (-47.301, 22.7477) (-46.962, 22.7477) knots 0 0 0 0 1 1 1 1
  spline S964 degree 3 poles (-46.962, 22.7477) (-47.4353, 21.0754) (-47.908, 19.4111) (-48.4577, 17.7622) knots 0 0 0 0 1 1 1 1
  spline S965 degree 3 poles (-48.4577, 17.7622) (-48.7867, 17.7622) (-49.1158, 17.7622) (-49.4548, 17.7622) knots 0 0 0 0 1 1 1 1
  spline S966 degree 3 poles (-49.4548, 17.7622) (-49.6193, 16.775) (-49.7838, 15.7879) (-49.9533, 14.7708) knots 0 0 0 0 1 1 1 1
  spline S967 degree 3 poles (-49.9533, 14.7708) (-50.4524, 16.4214) (-50.5035, 17.9121) (-50.4831, 19.6317) knots 0 0 0 0 1 1 1 1
  spline S968 degree 3 poles (-50.4831, 19.6317) (-50.4786, 20.1227) (-50.4741, 20.6137) (-50.4694, 21.1196) knots 0 0 0 0 1 1 1 1
  spline S969 degree 3 poles (-50.4694, 21.1196) (-50.4636, 21.4924) (-50.4579, 21.8651) (-50.4519, 22.2492) knots 0 0 0 0 1 1 1 1
  spline S970 degree 3 poles (-50.4519, 22.2492) (-49.9583, 22.0846) (-49.4648, 21.9201) (-48.9562, 21.7506) knots 0 0 0 0 1 1 1 1
  spline S971 degree 3 poles (-48.9562, 21.7506) (-48.6272, 22.0796) (-48.2981, 22.4087) (-47.9591, 22.7477) knots 0 0 0 0 1 1 1 1
  spline S972 degree 3 poles (43.7752, -8.1628) (44.5765, -9.7654) (44.3024, -11.3715) (44.2737, -13.1483) knots 0 0 0 0 1 1 1 1
  spline S973 degree 3 poles (44.2737, -13.1483) (41.8059, -13.1483) (39.338, -13.1483) (36.7954, -13.1483) knots 0 0 0 0 1 1 1 1
  spline S974 degree 3 poles (36.7954, -13.1483) (36.7954, -12.8193) (36.7954, -12.4902) (36.7954, -12.1512) knots 0 0 0 0 1 1 1 1
  spline S975 degree 3 poles (36.7954, -12.1512) (38.6052, -12.1512) (40.4149, -12.1512) (42.2795, -12.1512) knots 0 0 0 0 1 1 1 1
  spline S976 degree 3 poles (42.2795, -12.1512) (42.2795, -11.3286) (42.2795, -10.506) (42.2795, -9.6584) knots 0 0 0 0 1 1 1 1
  spline S977 degree 3 poles (42.2795, -9.6584) (43.0274, -8.7548) (43.0274, -8.7548) (43.7752, -8.1628) knots 0 0 0 0 1 1 1 1
  spline S978 degree 3 poles (-9.5703, 7.791) (-9.2413, 7.791) (-8.9122, 7.791) (-8.5732, 7.791) knots 0 0 0 0 1 1 1 1
  spline S979 degree 3 poles (-8.5732, 7.791) (-8.8758, 4.462) (-9.9573, 1.4587) (-11.066, -1.6815) knots 0 0 0 0 1 1 1 1
  spline S980 degree 3 poles (-11.066, -1.6815) (-11.2305, -1.6815) (-11.395, -1.6815) (-11.5645, -1.6815) knots 0 0 0 0 1 1 1 1
  spline S981 degree 3 poles (-11.5645, -1.6815) (-12.4078, 1.9984) (-11.3339, 4.5351) (-9.5703, 7.791) knots 0 0 0 0 1 1 1 1
  spline S982 degree 3 poles (-3.5876, 12.7766) (-2.765, 12.7766) (-1.9424, 12.7766) (-1.0949, 12.7766) knots 0 0 0 0 1 1 1 1
  spline S983 degree 3 poles (-1.0949, 12.7766) (-1.4239, 12.4475) (-1.7529, 12.1185) (-2.092, 11.7795) knots 0 0 0 0 1 1 1 1
  spline S984 degree 3 poles (-2.092, 11.7795) (-2.221, 10.1023) (-2.2747, 8.4459) (-2.2867, 6.7647) knots 0 0 0 0 1 1 1 1
  spline S985 degree 3 poles (-2.2867, 6.7647) (-2.347, 4.9451) (-2.4408, 3.9867) (-3.6071, 2.5523) knots 0 0 0 0 1 1 1 1
  spline S986 degree 3 poles (-3.6071, 2.5523) (-3.9297, 2.3068) (-4.2523, 2.0613) (-4.5847, 1.8084) knots 0 0 0 0 1 1 1 1
  spline S987 degree 3 poles (-4.5847, 1.8084) (-5.0833, 2.8055) (-5.0833, 2.8055) (-4.8048, 3.6916) knots 0 0 0 0 1 1 1 1
  spline S988 degree 3 poles (-4.8048, 3.6916) (-4.5879, 4.2247) (-4.5879, 4.2247) (-4.3666, 4.7685) knots 0 0 0 0 1 1 1 1
  spline S989 degree 3 poles (-4.3666, 4.7685) (-3.405, 7.4524) (-3.4453, 9.9569) (-3.5876, 12.7766) knots 0 0 0 0 1 1 1 1
  spline S990 degree 3 poles (6.3835, 14.7708) (6.1117, 11.2375) (5.0827, 8.1261) (3.8907, 4.7997) knots 0 0 0 0 1 1 1 1
  spline S991 degree 3 poles (3.8907, 4.7997) (3.7262, 4.7997) (3.5617, 4.7997) (3.3922, 4.7997) knots 0 0 0 0 1 1 1 1
  spline S992 degree 3 poles (3.3922, 4.7997) (3.5755, 7.9419) (3.9736, 10.4496) (5.3864, 13.2751) knots 0 0 0 0 1 1 1 1
  spline S993 degree 3 poles (5.3864, 13.2751) (4.2347, 13.2751) (3.083, 13.2751) (1.8965, 13.2751) knots 0 0 0 0 1 1 1 1
  spline S994 degree 3 poles (1.8965, 13.2751) (3.5257, 14.3613) (4.4294, 14.7708) (6.3835, 14.7708) knots 0 0 0 0 1 1 1 1
  spline S995 degree 3 poles (27.3228, 47.6755) (29.5281, 47.0017) (30.5716, 46.1314) (31.8098, 44.1856) knots 0 0 0 0 1 1 1 1
  spline S996 degree 3 poles (31.8098, 44.1856) (32.1838, 42.5342) (32.1838, 42.5342) (32.3084, 41.1943) knots 0 0 0 0 1 1 1 1
  spline S997 degree 3 poles (32.3084, 41.1943) (30.6277, 41.7545) (30.5341, 41.928) (29.7533, 43.4066) knots 0 0 0 0 1 1 1 1
  spline S998 degree 3 poles (29.7533, 43.4066) (29.5875, 43.7145) (29.4217, 44.0223) (29.2508, 44.3395) knots 0 0 0 0 1 1 1 1
  spline S999 degree 3 poles (29.2508, 44.3395) (28.9372, 44.9512) (28.6274, 45.565) (28.32, 46.1798) knots 0 0 0 0 1 1 1 1
  spline S1000 degree 3 poles (28.32, 46.1798) (27.9909, 46.1798) (27.6619, 46.1798) (27.3228, 46.1798) knots 0 0 0 0 1 1 1 1
  spline S1001 degree 3 poles (27.3228, 46.1798) (27.3228, 46.6734) (27.3228, 47.167) (27.3228, 47.6755) knots 0 0 0 0 1 1 1 1
  spline S1002 degree 3 poles (-12.7486, 48.7038) (-12.2203, 48.7004) (-12.2203, 48.7004) (-11.6814, 48.697) knots 0 0 0 0 1 1 1 1
  spline S1003 degree 3 poles (-11.6814, 48.697) (-10.8115, 48.6911) (-9.9416, 48.6821) (-9.0717, 48.6726) knots 0 0 0 0 1 1 1 1
  spline S1004 degree 3 poles (-9.0717, 48.6726) (-8.9072, 48.0145) (-8.7427, 47.3564) (-8.5732, 46.6784) knots 0 0 0 0 1 1 1 1
  spline S1005 degree 3 poles (-8.5732, 46.6784) (-9.0668, 46.4316) (-9.0668, 46.4316) (-9.5703, 46.1798) knots 0 0 0 0 1 1 1 1
  spline S1006 degree 3 poles (-9.5703, 46.1798) (-9.5703, 46.6734) (-9.5703, 47.167) (-9.5703, 47.6755) knots 0 0 0 0 1 1 1 1